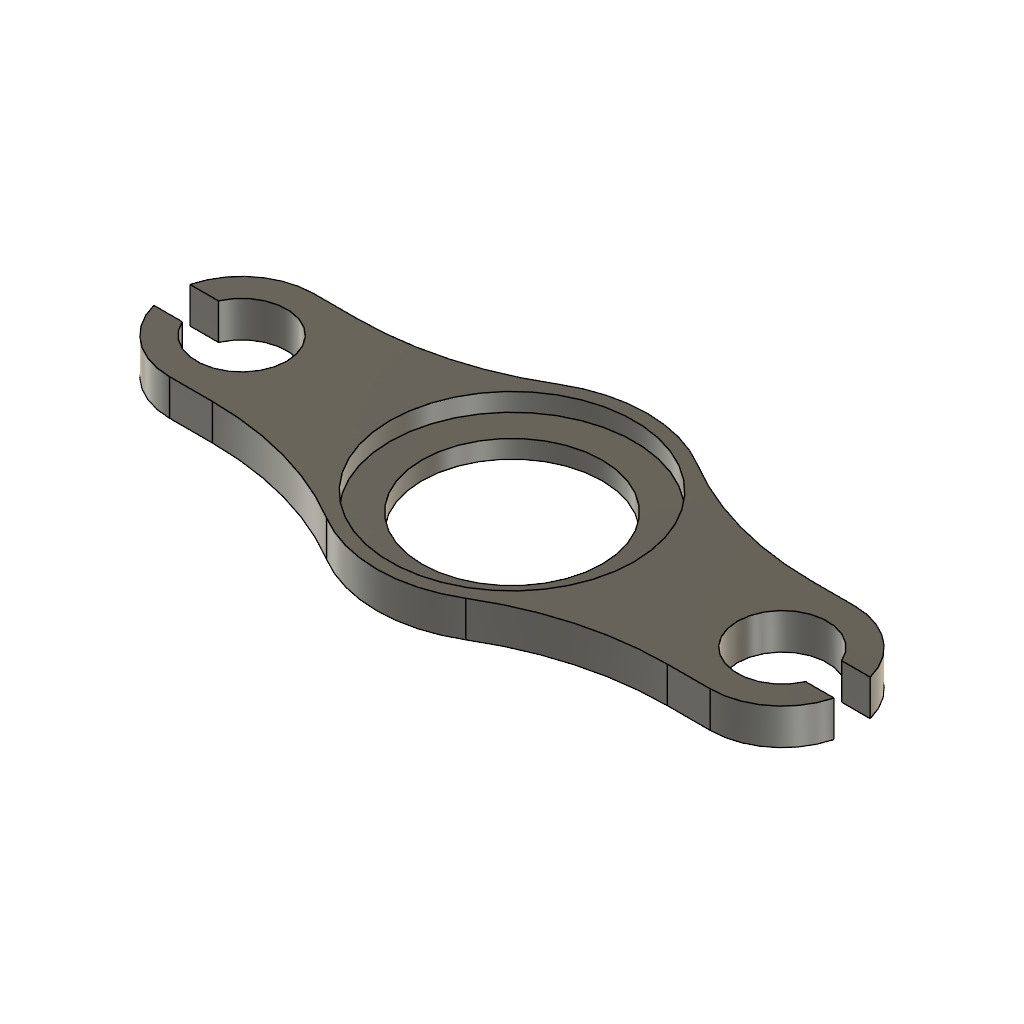
exercise 7 (Autodesk Fusion 360 design; units mm, degrees)
part number: 2026-10-03-23-49-57-812
Autodesk Fusion 360 part; units mm, degrees
sketch "Sketch1" plane through (0, 0, 0) normal (0, 0, 1) x (1, 0, 0)
  circle A0 centre (0, 0) radius 67.8
  circle A1 centre (0, 0) radius 50
  line L0 (-150, 40) -> (-126.1943, 40)
  line L1 (-150, -40) -> (-126.1943, -40)
  line L2 (150, 40) -> (126.1943, 40)
  line L3 (150, -40) -> (126.1943, -40)
  arc A2 (-38.6309, -64.2857) -> (38.6309, -64.2857) centre (0, 0) ccw
  arc A3 (38.6309, 64.2857) -> (-38.6309, 64.2857) centre (0, 0) ccw
  line L4 (-172.9129, 10) -> (-188.7298, 10)
  line L5 (-172.9129, -10) -> (-188.7298, -10)
  arc A4 (-172.9129, -10) -> (-172.9129, 10) centre (-150, 0) ccw
  arc A5 (-150, 40) -> (-188.7298, 10) centre (-150, 0) ccw
  arc A6 (-188.7298, -10) -> (-150, -40) centre (-150, 0) ccw
  line L6 (188.7298, 10) -> (172.9129, 10)
  line L7 (188.7298, -10) -> (172.9129, -10)
  arc A7 (172.9129, 10) -> (172.9129, -10) centre (150, 0) ccw
  arc A8 (150, -40) -> (188.7298, -10) centre (150, 0) ccw
  arc A9 (188.7298, 10) -> (150, 40) centre (150, 0) ccw
  arc A10 (-126.1943, 40) -> (-38.6309, 64.2857) centre (-126.1943, 210) ccw
  arc A11 (-38.6309, -64.2857) -> (-126.1943, -40) centre (-126.1943, -210) ccw
  arc A12 (38.6309, 64.2857) -> (126.1943, 40) centre (126.1943, 210) ccw
  arc A13 (126.1943, -40) -> (38.6309, -64.2857) centre (126.1943, -210) ccw
  dimension "d1" = 135.6
  dimension "d2" = 100
  dimension "d3" = 50
  dimension "d4" = 50
  dimension "d5" = 150
  dimension "d6" = 150
  dimension "d7" = 150
  dimension "d8" = 80
  dimension "d9" = 80
  dimension "d16" = 170
  dimension "d17" = 170
  dimension "d18" = 170
  constraint coincident A0.centre A1.centre
  constraint concentric A0 A1
  constraint concentric A0 A2
  constraint concentric A4 A5
  constraint concentric A7 A8
  constraint tangent L0 A5
  constraint horizontal L0
  constraint tangent L1 A6
  constraint horizontal L1
  constraint tangent L2 A9
  constraint horizontal L2
  constraint tangent L3 A8
  constraint parallel L0 L3
  constraint concentric A2 A3
  constraint horizontal L4
  constraint concentric A5 A6
  constraint horizontal L6
  constraint horizontal L7
  constraint concentric A8 A9
  constraint tangent L0 A10
  constraint tangent A3 A10
  constraint tangent A2 A11
  constraint tangent L1 A11
  constraint tangent A3 A12
  constraint tangent L2 A12
  constraint tangent L3 A13
  constraint tangent A2 A13
  constraint equal A12 A13
  measures "d1" diameter of A0
  measures "d2" diameter of A1
  measures "d3" diameter of A7
  measures "d4" diameter of A4
  measures "d5" distance of A0.centre A4.centre
  measures "d6" distance of A0.centre A7.centre
  measures "d7" diameter of A2
  measures "d8" diameter of A5
  measures "d9" diameter of A8
  measures "d16" radius of A10
  measures "d17" radius of A11
  measures "d18" radius of A12
extrude "Extrude1" add sketch "Sketch1" along normal blind 20 contours L0 L1 L2 L3 A2 A3 L4 L5 A4 A5 A6 L6 L7 A7 A8 A9 A10 A11 A12 A13
extrude "Extrude2" add sketch "Sketch1" along normal blind 10 contours A0
